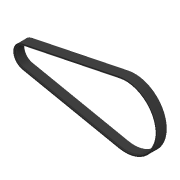
# Autodesk Inventor part: Tandriem16naar60T
Saved by Autodesk Inventor 2020.3 (Build 243373000, 373)
## iProperties
Created: 2020-05-14
Part Number: Tandriem16naar60T
Material: Rubber
Document SubType Name: Modeling
Designer: Svend
Density: 0.93 g/cm^3
Appearance: Rubber - Black
Author: Svend
Autodesk Inventor part; units mm, degrees
ref_plane "YZ Plane" through (0, 0, 0) normal (1, 0, 0) x (0, 1, 0)
ref_plane "XZ Plane" through (0, 0, 0) normal (0, 1, 0) x (-1, 0, 0)
ref_plane "XY Plane" through (0, 0, 0) normal (0, 0, 1) x (1, 0, 0)
sketch "Sketch1" plane through (0, 0, 0) normal (0, 0, 1) x (1, 0, 0)
  arc A0 (-1.2105, 5.8766) -> (-1.2105, -5.8766) centre (0, 0) ccw
  arc A1 (59.8885, -18.4624) -> (59.8885, 18.4624) centre (63.6915, 0) ccw
  line L0 (-1.2105, 5.8766) -> (59.8885, 18.4624)
  line L1 (-1.2105, -5.8766) -> (59.8885, -18.4624)
  line L2 (59.6262, 19.7356) -> (-1.4728, 7.1499)
  arc A2 (-1.4728, 7.1499) -> (-1.4728, -7.1499) centre (0, 0) ccw
  line L3 (-1.4728, -7.1499) -> (59.6262, -19.7356)
  arc A3 (59.6262, -19.7356) -> (59.6262, 19.7356) centre (63.6915, 0) ccw
  dimension "d0" = 12
  dimension "d1" = 37.7
  dimension "d3" = 1.3
  dimension "d9" = 63.6915
  constraints: 8 end point, 8 point on circle, 4 centre point, 4 tangent, 1 coincident, 1 horizontal alignment, 3 other
  measures "d0" diameter of A0
  measures "d1" diameter of A1
  measures "d3" distance between parallel lines of L0 L2
  measures "d9" distance of A1.centre A0.centre
extrude "Extrusion1" add sketch "Sketch1" along normal mid plane 6
chamfer "Chamfer1" distance 0.5 angle 45 8 edges at (-6, 0, 3) (29.339, 12.1695, 3) (82.5415, 0, 3) (29.339, -12.1695, 3) (-6, 0, -3) (29.339, -12.1695, -3) (82.5415, 0, -3) (29.339, 12.1695, -3)
body "Solid1"
